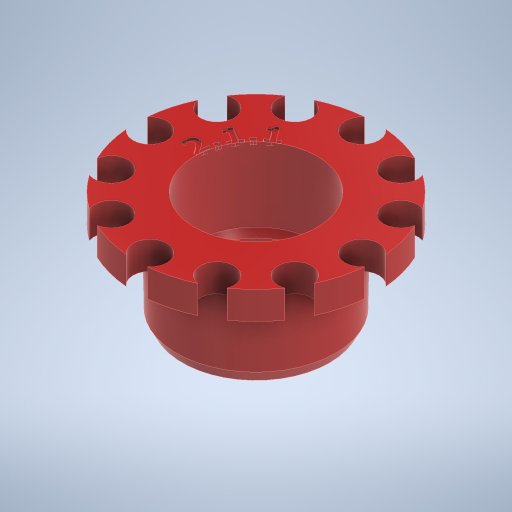
# Autodesk Inventor part: WindTowerNacelleInterface
Saved by Autodesk Inventor 2024.3 (Build 283343000, 343)
## iProperties
Created: 2024-11-20
Part Number: WindTowerNacelleInterface
Material: PET-Kunststoff
Document SubType Name: Modeling
Designer: Maximilian Hock
Density: 1.541 g/cm^3
Appearance: Rot
Author: Maximilian Hock
## iProperties of the stored document WindTowerNacelleInterface_3D-Druck.ipt
Created: 2024-12-16
Part Number: WindTowerNacelleInterface_3D-Druck
Material: Generisch
Document SubType Name: Modeling
Designer: Maximilian Hock
Density: 1 g/cm^3
Appearance: Vorgabe
Author: Maximilian Hock
Autodesk Inventor part; units mm, degrees
ref_plane "YZ Plane" through (0, 0, 0) normal (1, 0, 0) x (0, 1, 0)
ref_plane "XZ Plane" through (0, 0, 0) normal (0, 1, 0) x (-1, 0, 0)
ref_plane "XY Plane" through (0, 0, 0) normal (0, 0, 1) x (1, 0, 0)
sketch "Skizze1" plane through (0, 0, 0) normal (0, 0, 1) x (1, 0, 0)
  circle A0 centre (0, 0) radius 14.5
  dimension "d0" = 29
  constraints: 1 centre point, 1 coincident
  measures "d0" diameter of A0
extrude "Extrusion1" add sketch "Skizze1" along normal blind 15
sketch "Skizze2" plane through (0, 0, 15) normal (0, 0, 1) x (1, 0, 0)
  circle A0 centre (0, 0) radius 14.5 projected
  circle A1 centre (0, 0) radius 21.5
  dimension "d3" = 7
  constraints: 1 centre point
  measures "d3" radial gap between concentric circles of A0 A1
extrude "Extrusion2" add sketch "Skizze2" along normal blind 5 contours A0 | A1
sketch "Skizze6" plane through (0, 0, 20) normal (0, 0, 1) x (1, 0, 0)
  circle A0 centre (0, 19.05) radius 3.05
  circle A1 centre (0, 0) radius 16 construction
  dimension "d19" = 32
  dimension "d21" = 6.1
  constraints: 2 centre point, 1 coincident, 1 tangent, 1 vertical alignment
  measures "d19" diameter of A1
  measures "d21" diameter of A0
extrude "Extrusion6" cut sketch "Skizze6" against normal through all
sketch "Skizze8" plane through (0, 0, 20) normal (0, 0, 1) x (1, 0, 0)
  point P0 (0, 0)
  point P1 (0, 0)
  constraints: 1 coincident
hole "Bohrung1" at (0, 0, 20) direction (0, 0, -1) diameter 20.1 end through all counterbore diameter 22.1 counterbore depth 13.3
pattern_circular "Runde Anordnung1" count 12 over 360 about axis through (0, 0, -10) along (0, 0, 1) of "Extrusion6"
chamfer "Fasen1" distance 1 angle 45 1 edges at (0, 10.05, 6.7)
chamfer "Fasen2" distance 15 angle 1 1 edges at (-14.5, 0, 0) measured on face at (14.453, -1.1668, 10)
chamfer "Fasen3" distance 1 distance2 2 1 edges at (-14.2383, 0, 0) measured on face at (12.6798, -1.5396, 0)
sketch "Skizze9" plane through (0, 0, 20) normal (0, 0, 1) x (1, 0, 0)
  arc A0 (9.0371, 19.5085) -> (12.3763, 17.5806) centre (9.525, 16.4978) ccw projected
  arc A1 (9.0371, 19.5085) -> (1.9279, 21.4134) centre (0, 0) ccw projected
  arc A2 (-1.9279, 21.4134) -> (1.9279, 21.4134) centre (0, 19.05) ccw projected
  arc A3 (-1.9279, 21.4134) -> (-9.0371, 19.5085) centre (0, 0) ccw projected
  arc A4 (-12.3763, 17.5806) -> (-9.0371, 19.5085) centre (-9.525, 16.4978) ccw projected
  arc A5 (-12.3763, 17.5806) -> (-17.5806, 12.3763) centre (0, 0) ccw projected
  arc A6 (-19.5085, 9.0371) -> (-17.5806, 12.3763) centre (-16.4978, 9.525) ccw projected
  arc A7 (-19.5085, 9.0371) -> (-21.4134, 1.9279) centre (0, 0) ccw projected
  arc A8 (-21.4134, -1.9279) -> (-21.4134, 1.9279) centre (-19.05, 0) ccw projected
  arc A9 (-21.4134, -1.9279) -> (-19.5085, -9.0371) centre (0, 0) ccw projected
  arc A10 (-17.5806, -12.3763) -> (-19.5085, -9.0371) centre (-16.4978, -9.525) ccw projected
  arc A11 (-17.5806, -12.3763) -> (-12.3763, -17.5806) centre (0, 0) ccw projected
  arc A12 (-9.0371, -19.5085) -> (-12.3763, -17.5806) centre (-9.525, -16.4978) ccw projected
  arc A13 (-9.0371, -19.5085) -> (-1.9279, -21.4134) centre (0, 0) ccw projected
  arc A14 (1.9279, -21.4134) -> (-1.9279, -21.4134) centre (0, -19.05) ccw projected
  arc A15 (1.9279, -21.4134) -> (9.0371, -19.5085) centre (0, 0) ccw projected
  arc A16 (12.3763, -17.5806) -> (9.0371, -19.5085) centre (9.525, -16.4978) ccw projected
  arc A17 (12.3763, -17.5806) -> (17.5806, -12.3763) centre (0, 0) ccw projected
  arc A18 (19.5085, -9.0371) -> (17.5806, -12.3763) centre (16.4978, -9.525) ccw projected
  arc A19 (19.5085, -9.0371) -> (21.4134, -1.9279) centre (0, 0) ccw projected
  arc A20 (21.4134, 1.9279) -> (21.4134, -1.9279) centre (19.05, 0) ccw projected
  arc A21 (21.4134, 1.9279) -> (19.5085, 9.0371) centre (0, 0) ccw projected
  arc A22 (17.5806, 12.3763) -> (19.5085, 9.0371) centre (16.4978, 9.525) ccw projected
  arc A23 (17.5806, 12.3763) -> (12.3763, 17.5806) centre (0, 0) ccw projected
  circle A24 centre (0, 0) radius 11.05 projected
  line L0 (-10.7536, 2.8993) -> (-11.1071, 0.3512)
  line L1 (-11.1071, 0.3512) -> (-11.6718, 0.4295)
  spline S0 degree 2 poles (-11.6718, 0.4295) (-11.8854, 0.7885) (-12.2689, 1.3685) (-12.447, 1.5908) knots 0 0 0 1 2 2 2
  spline S1 degree 2 poles (-12.447, 1.5908) (-12.6785, 1.8835) (-13.0543, 2.1676) (-13.2678, 2.1972) knots 0 0 0 1 2 2 2
  spline S2 degree 2 poles (-13.2678, 2.1972) (-13.5094, 2.2307) (-13.808, 1.9772) (-13.8439, 1.7188) knots 0 0 0 1 2 2 2
  spline S3 degree 2 poles (-13.8439, 1.7188) (-13.8622, 1.5867) (-13.8303, 1.3418) (-13.7965, 1.2139) knots 0 0 0 1 2 2 2
  spline S4 degree 2 poles (-13.7965, 1.2139) (-13.7595, 1.0885) (-13.6705, 0.9044) (-13.6482, 0.8583) knots 0 0 0 1 2 2 2
  line L2 (-13.6482, 0.8583) -> (-13.6576, 0.7909)
  line L3 (-13.6576, 0.7909) -> (-14.4133, 0.8958)
  spline S5 degree 2 poles (-14.4133, 0.8958) (-14.4633, 1.0516) (-14.5228, 1.6956) (-14.4827, 1.9849) knots 0 0 0 1 2 2 2
  spline S6 degree 2 poles (-14.4827, 1.9849) (-14.397, 2.603) (-13.7582, 3.1615) (-13.261, 3.0925) knots 0 0 0 1 2 2 2
  spline S7 degree 2 poles (-13.261, 3.0925) (-12.9547, 3.05) (-12.4049, 2.6788) (-12.1142, 2.2977) knots 0 0 0 1 2 2 2
  spline S8 degree 2 poles (-12.1142, 2.2977) (-11.9355, 2.0582) (-11.6674, 1.6172) (-11.612, 1.5208) knots 0 0 0 1 2 2 2
  line L4 (-11.612, 1.5208) -> (-11.4082, 2.9901)
  line L5 (-11.4082, 2.9901) -> (-10.7536, 2.8993)
  line L6 (-10.2645, 4.1127) -> (-10.5445, 3.3302)
  line L7 (-10.5445, 3.3302) -> (-11.4151, 3.6417)
  line L8 (-11.4151, 3.6417) -> (-11.1351, 4.4242)
  line L9 (-11.1351, 4.4242) -> (-10.2645, 4.1127)
  line L10 (-8.7774, 6.8259) -> (-9.9845, 4.8544)
  line L11 (-9.9845, 4.8544) -> (-10.5045, 5.1729)
  line L12 (-10.5045, 5.1729) -> (-10.1195, 5.8018)
  line L13 (-10.1195, 5.8018) -> (-11.699, 6.7689)
  line L14 (-11.699, 6.7689) -> (-12.0841, 6.14)
  line L15 (-12.0841, 6.14) -> (-12.5703, 6.4377)
  spline S9 degree 2 poles (-12.5703, 6.4377) (-12.4859, 6.5756) (-12.3548, 6.8711) (-12.3431, 6.977) knots 0 0 0 1 2 2 2
  spline S10 degree 2 poles (-12.3431, 6.977) (-12.3337, 7.101) (-12.4306, 7.3067) (-12.5457, 7.3904) knots 0 0 0 1 2 2 2
  line L16 (-12.5457, 7.3904) -> (-12.1458, 8.0435)
  line L17 (-12.1458, 8.0435) -> (-9.6737, 6.5299)
  line L18 (-9.6737, 6.5299) -> (-9.2975, 7.1443)
  line L19 (-9.2975, 7.1443) -> (-8.7774, 6.8259)
  line L20 (-7.7623, 7.8753) -> (-8.3319, 7.2702)
  line L21 (-8.3319, 7.2702) -> (-9.0052, 7.9039)
  line L22 (-9.0052, 7.9039) -> (-8.4356, 8.5091)
  line L23 (-8.4356, 8.5091) -> (-7.7623, 7.8753)
  line L24 (-5.314, 9.7671) -> (-7.2089, 8.4431)
  line L25 (-7.2089, 8.4431) -> (-7.5582, 8.943)
  line L26 (-7.5582, 8.943) -> (-6.9537, 9.3654)
  line L27 (-6.9537, 9.3654) -> (-8.0145, 10.8836)
  line L28 (-8.0145, 10.8836) -> (-8.619, 10.4612)
  line L29 (-8.619, 10.4612) -> (-8.9455, 10.9286)
  spline S11 degree 2 poles (-8.9455, 10.9286) (-8.813, 11.0212) (-8.5746, 11.2396) (-8.5216, 11.332) knots 0 0 0 1 2 2 2
  spline S12 degree 2 poles (-8.5216, 11.332) (-8.4634, 11.4419) (-8.4699, 11.6691) (-8.5419, 11.7919) knots 0 0 0 1 2 2 2
  line L30 (-8.5419, 11.7919) -> (-7.9141, 12.2305)
  line L31 (-7.9141, 12.2305) -> (-6.2539, 9.8543)
  line L32 (-6.2539, 9.8543) -> (-5.6633, 10.267)
  line L33 (-5.6633, 10.267) -> (-5.314, 9.7671)
  constraints: 1 other
emboss "Prägen1" sketch "Skizze9" operation cut depth 0.5 direction (0, 0, -1) contours L0 L1 S0 S1 S2 S3 S4 L2 L3 S5 S6 S7 S8 L4 L5 | L6 L7 L8 L9 | L10 L11 L12 L13 L14 L15 S9 S10 L16 L17 L18 L19 | L20 L21 L22 L23 | L24 L25 L26 L27 L28 L29 S11 S12 L30 L31 L32 L33
equation "\"d0\" = WindTowerInnerDiameter"
equation "\"d19\" = WindTowerOuterDiameter"
equation "\"d21\" = AxleDiameter + Clearance"
equation "\"d26\" = BearingOuterDiameter + Clearance"
equation "\"d27\" = 1.9 * BearingHeight"
equation "\"WindTowerInnerDiameter\" = 29"
equation "\"WindTowerOuterDiameter\" = 32"
equation "\"AxleDiameter\" = 6"
equation "\"Clearance\" = 0.1"
equation "\"BearingOuterDiameter\" = 22"
equation "\"BearingHeight\" = 7"
